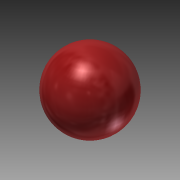
# Autodesk Inventor part: ESFERA_6MM
Saved by Autodesk Inventor 2015 (Build 190159000, 159)
## iProperties
Created: 2016-03-03
Part Number: ESFERA_6MM
Material: Generic
Document SubType Name: Modeling
Designer: Everton
Density: 1 g/cm^3
Appearance: Default
Author: Everton
Autodesk Inventor part; units mm, degrees
ref_plane "YZ Plane" through (0, 0, 0) normal (1, 0, 0) x (0, 1, 0)
ref_plane "XZ Plane" through (0, 0, 0) normal (0, 1, 0) x (-1, 0, 0)
ref_plane "XY Plane" through (0, 0, 0) normal (0, 0, 1) x (1, 0, 0)
sketch "Sketch1" plane through (0, 0, 0) normal (0, 1, 0) x (-1, 0, 0)
  arc A0 (4.4274, -13.723) -> (4.4274, -7.723) centre (4.4274, -10.723) ccw
  line L0 (4.4274, -7.723) -> (4.4274, -13.723)
  point P0 (0, 0)
  dimension "d0" = 6
  constraints: 2 end point, 2 point on circle, 1 centre point, 1 vertical
  measures "d0" diameter of A0
revolve "Revolution1" add sketch "Sketch1" angle 360 about axis through (-4.4274, 0, -7.723) along (0, 0, -1)
body "Solid1"
